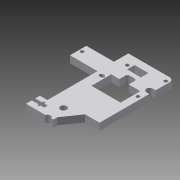
# Autodesk Inventor part: yCarTopper
Saved by Autodesk Inventor 2013 (Build 170138000, 138)
## iProperties
Created: 2015-01-14
Part Number: yCarTopper
Material: Generic
Document SubType Name: Modeling
Designer: dzban
Density: 1 g/cm^3
Author: dzban
Autodesk Inventor part; units mm, degrees
ref_plane "YZ Plane" through (0, 0, 0) normal (1, 0, 0) x (0, 1, 0)
ref_plane "XZ Plane" through (0, 0, 0) normal (0, 1, 0) x (-1, 0, 0)
ref_plane "XY Plane" through (0, 0, 0) normal (0, 0, 1) x (1, 0, 0)
sketch "Sketch1" plane through (0, 0, 0) normal (0, 0, 1) x (1, 0, 0)
  arc A0 (0, 83) -> (-4, 87) centre (-4, 83) ccw
  line L0 (-39.2369, 87) -> (-4, 87)
  line L1 (-39.2369, 74.6) -> (-39.2369, 87)
  line L2 (-63, 74.6) -> (-39.2369, 74.6)
  line L3 (-63, 60.5) -> (-63, 74.6)
  line L4 (-39.3408, 60.5) -> (-63, 60.5)
  line L5 (-39.3408, 17.4533) -> (-39.3408, 60.5)
  line L6 (-45.8408, 17.4533) -> (-39.3408, 17.4533)
  line L7 (-45.8408, 13.4533) -> (-45.8408, 17.4533)
  line L8 (-39.8408, 13.4533) -> (-45.8408, 13.4533)
  line L9 (-39.8408, 14.7033) -> (-39.8408, 13.4533)
  line L10 (-38.0408, 14.7033) -> (-39.8408, 14.7033)
  line L11 (-38.0408, 13.4533) -> (-38.0408, 14.7033)
  line L12 (-35.0408, 13.4533) -> (-38.0408, 13.4533)
  line L13 (-35.0408, 10.4533) -> (-35.0408, 13.4533)
  line L14 (-38.0408, 10.4533) -> (-35.0408, 10.4533)
  line L15 (-38.0408, 9.2033) -> (-38.0408, 10.4533)
  line L16 (-39.8408, 9.2033) -> (-38.0408, 9.2033)
  line L17 (-39.8408, 10.4533) -> (-39.8408, 9.2033)
  line L18 (-45.8408, 10.4533) -> (-39.8408, 10.4533)
  line L19 (-45.8408, 5.4533) -> (-45.8408, 10.4533)
  line L20 (-29.0795, 5.4533) -> (-45.8408, 5.4533)
  arc A1 (-23.9205, 5.4533) -> (-29.0795, 5.4533) centre (-26.5, 4.5) ccw
  line L21 (-22.2439, 5.4533) -> (-23.9205, 5.4533)
  line L22 (-22.2439, 8.8497) -> (-22.2439, 5.4533)
  line L23 (-12.4378, 23) -> (-22.2439, 8.8497)
  line L24 (0, 23) -> (-12.4378, 23)
  line L25 (0, 65.75) -> (0, 23)
  line L26 (-2.5, 65.75) -> (0, 65.75)
  arc A2 (-2.5, 71.25) -> (-2.5, 65.75) centre (-2.5, 68.5) ccw
  line L27 (0, 71.25) -> (-2.5, 71.25)
  line L28 (0, 83) -> (0, 71.25)
  line L29 (-27.9, 74.6) -> (-27.9, 81)
  line L30 (-27.9, 81) -> (-16, 81)
  line L31 (-16, 81) -> (-16, 74.6)
  line L32 (-16, 74.6) -> (-27.9, 74.6)
  circle A3 centre (-26.5, 18.5) radius 2.75
  line L33 (-34.7, 60.5) -> (-33.3, 60.5)
  arc A4 (-33.3, 57.5) -> (-33.3, 60.5) centre (-33.3, 59) ccw
  line L34 (-33.3, 57.5) -> (-34.7, 57.5)
  arc A5 (-34.7, 60.5) -> (-34.7, 57.5) centre (-34.7, 59) ccw
  circle A6 centre (-30.9, 77.8) radius 1.5
  circle A7 centre (-3, 59) radius 1.5
  circle A8 centre (-2.5, 82.5) radius 1.5
  circle A9 centre (-60.5, 68.5) radius 1.5
  line L35 (-31, 64) -> (-31, 47)
  line L36 (-24, 64) -> (-31, 64)
  line L37 (-24, 69) -> (-24, 64)
  arc A10 (-22, 71) -> (-24, 69) centre (-22, 69) ccw
  line L38 (-18, 71) -> (-22, 71)
  arc A11 (-16, 69) -> (-18, 71) centre (-18, 69) ccw
  line L39 (-16, 64) -> (-16, 69)
  line L40 (-6, 64) -> (-16, 64)
  line L41 (-6, 47) -> (-6, 64)
  line L42 (-31, 47) -> (-6, 47)
  point P0 (0, 0)
  constraints: 86 end point, 14 point on circle, 12 centre point
extrude "Extrusion1" add sketch "Sketch1" along normal blind 6
body "Solid1"
